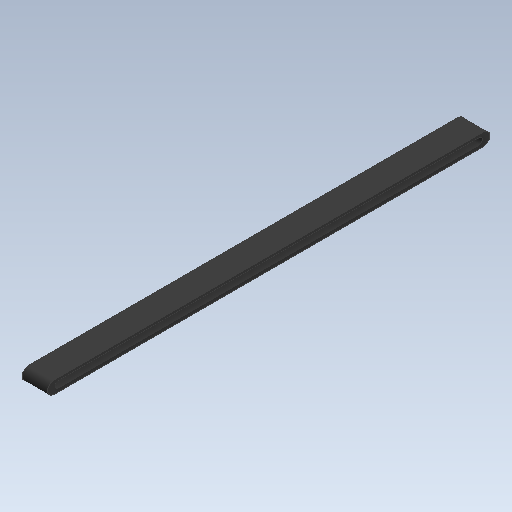
# Autodesk Inventor part: belt
Saved by Autodesk Inventor 2020 (Build 240168000, 168)
## iProperties
Created: 2021-07-09
Part Number: belt
Material: Rubber
Document SubType Name: Modeling
Designer: pc
Density: 0.93 g/cm^3
Appearance: Rubber - Black
Author: pc
Autodesk Inventor part; units mm, degrees
ref_plane "YZ Plane" through (0, 0, 0) normal (1, 0, 0) x (0, 1, 0)
ref_plane "XZ Plane" through (0, 0, 0) normal (0, 1, 0) x (-1, 0, 0)
ref_plane "XY Plane" through (0, 0, 0) normal (0, 0, 1) x (1, 0, 0)
sketch "Sketch1" plane through (0, 0, 0) normal (1, 0, 0) x (0, 1, 0)
  line L0 (137.9553, -481.4639) -> (137.9553, 382.1361)
  line L1 (112.5553, 382.1361) -> (112.5553, -481.4639)
  arc A0 (137.9553, 382.1361) -> (112.5553, 382.1361) centre (125.2553, 382.1361) ccw
  arc A1 (112.5553, -481.4639) -> (137.9553, -481.4639) centre (125.2553, -481.4639) ccw
  point P0 (0, 0)
  constraints: 4 end point, 4 point on circle, 4 tangent, 2 centre point, 1 parallel
extrude "Extrusion1" add sketch "Sketch1" along normal blind 50.8
sketch "Sketch2" plane through (50.8, 0, 0) normal (1, 0, 0) x (0, 0, -1)
  line L0 (-373.1211, 132.1899) -> (472.6989, 132.1899)
  line L1 (472.6989, 119.4899) -> (-373.1211, 119.4899)
  arc A0 (-373.1211, 132.1899) -> (-373.1211, 119.4899) centre (-373.1211, 125.8399) ccw
  arc A1 (472.6989, 119.4899) -> (472.6989, 132.1899) centre (472.6989, 125.8399) ccw
  point P0 (0, 0)
  constraints: 4 end point, 4 point on circle, 4 tangent, 2 centre point, 1 horizontal, 1 parallel
extrude "Extrusion2" cut sketch "Sketch2" against normal blind 50.8
body "Solid1"
